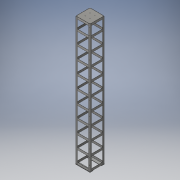
# Autodesk Inventor part: Celosia
Saved by Autodesk Inventor 2016 (Build 200138000, 138)
## iProperties
Created: 2017-01-18
Part Number: Celosia
Material: Generic
Document SubType Name: Modeling
Designer: admin
Density: 1 g/cm^3
Appearance: Default
Author: admin
Autodesk Inventor part; units mm, degrees
(part 1 of 3)
ref_plane "YZ Plane" through (0, 0, 0) normal (1, 0, 0) x (0, 1, 0)
ref_plane "XZ Plane" through (0, 0, 0) normal (0, 1, 0) x (-1, 0, 0)
ref_plane "XY Plane" through (0, 0, 0) normal (0, 0, 1) x (1, 0, 0)
sketch "Sketch1" plane through (0, 0, 0) normal (0, 1, 0) x (-1, 0, 0)
  line L0 (350, 345.4342) -> (345.4342, 350)
  line L1 (350, 320.2894) -> (342, 328.2894)
  line L2 (328.2894, 342) -> (320.2894, 350)
  line L3 (350, 295.1447) -> (342, 303.1447)
  line L4 (303.1447, 342) -> (295.1447, 350)
  line L5 (350, 270) -> (342, 278)
  line L6 (278, 342) -> (270, 350)
  line L7 (-270.2598, 345.6939) -> (-274.5658, 350)
  line L8 (-291.7106, 342) -> (-299.7106, 350)
  line L9 (-316.8553, 342) -> (-324.8553, 350)
  line L10 (-339.0697, 339.0697) -> (-350, 350)
  line L11 (-342, 316.8553) -> (-350, 324.8553)
  line L12 (-342, 291.7106) -> (-350, 299.7106)
  line L13 (-345.6939, 270.2598) -> (-350, 274.5658)
  line L14 (350, -273) -> (347, -270)
  line L15 (350, -298.1447) -> (342, -290.1447)
  line L16 (350, -323.2894) -> (342, -315.2894)
  line L17 (350, -348.4342) -> (339.6983, -338.1324)
  line L18 (326.4211, -350) -> (318.4211, -342)
  line L19 (301.2764, -350) -> (293.2764, -342)
  line L20 (276.1317, -350) -> (271.5658, -345.4342)
  line L21 (271.5658, -345.4342) -> (270.7161, -344.5844)
  line L22 (-270.3806, -345.0866) -> (-273.0153, -342.4519)
  line L23 (-342.4189, -273.0483) -> (-345.0146, -270.4526)
  line L24 (-290.6119, -350) -> (-298.6119, -342)
  line L25 (-342, -298.6119) -> (-350, -290.6119)
  line L26 (-315.7566, -350) -> (-323.7566, -342)
  line L27 (-342, -323.7566) -> (-350, -315.7566)
  line L28 (-340.9013, -350) -> (-350, -340.9013)
  line L29 (-310, 360) -> (-310, 342)
  line L30 (-319, 350) -> (-319, 342)
  line L31 (-301, 350) -> (-301, 342)
  line L32 (310, -360) -> (310, -342)
  line L33 (319, -350) -> (319, -342)
  line L34 (301, -350) -> (301, -342)
  line L35 (350, 270) -> (347, 270)
  line L36 (350, 350) -> (270, 350)
  line L37 (270, 350) -> (270, 347)
  line L38 (332, 342) -> (275, 342)
  line L39 (342, 332) -> (342, 275)
  line L40 (270, 347) -> (270.3806, 345.0866)
  line L41 (270.3806, 345.0866) -> (271.4645, 343.4645)
  line L42 (271.4645, 343.4645) -> (273.0866, 342.3806)
  line L43 (273.0866, 342.3806) -> (275, 342)
  line L44 (342, 275) -> (342.3806, 273.0866)
  line L45 (342.3806, 273.0866) -> (343.4645, 271.4645)
  line L46 (343.4645, 271.4645) -> (345.0866, 270.3806)
  line L47 (345.0866, 270.3806) -> (347, 270)
  line L48 (350, 350) -> (350, 270)
  line L49 (332, 342) -> (335.8268, 341.2388)
  arc A0 (341.2388, 335.8268) -> (335.8268, 341.2388) centre (332, 332) ccw
  line L50 (341.2388, 335.8268) -> (342, 332)
  line L51 (-347, 270) -> (-350, 270)
  line L52 (-270, 350) -> (-350, 350)
  line L53 (-350, 350) -> (-350, 270)
  line L54 (-347, 270) -> (-345.0866, 270.3806)
  line L55 (-345.0866, 270.3806) -> (-343.4645, 271.4645)
  line L56 (-343.4645, 271.4645) -> (-342.3806, 273.0866)
  line L57 (-342.3806, 273.0866) -> (-342, 275)
  line L58 (-275, 342) -> (-273.0866, 342.3806)
  line L59 (-273.0866, 342.3806) -> (-271.4645, 343.4645)
  line L60 (-271.4645, 343.4645) -> (-270.3806, 345.0866)
  line L61 (-270.3806, 345.0866) -> (-270, 347)
  line L62 (-270, 347) -> (-270, 350)
  line L63 (-275, 342) -> (-332, 342)
  line L64 (-342, 332) -> (-342, 275)
  line L65 (-342, 332) -> (-341.2388, 335.8268)
  arc A1 (-335.8268, 341.2388) -> (-341.2388, 335.8268) centre (-332, 332) ccw
  line L66 (-335.8268, 341.2388) -> (-332, 342)
  line L67 (270, 347) -> (270, 342)
  line L68 (-270, 347) -> (-270, 342)
  line L69 (-270, 342) -> (270, 342)
  line L70 (-270, 350) -> (270, 350)
  circle A2 centre (-330, -330) radius 7
  line L71 (-316, -330) -> (-344, -330)
  line L72 (-330, -316) -> (-330, -344)
  circle A3 centre (330, -330) radius 7
  line L73 (344, -330) -> (316, -330)
  line L74 (330, -316) -> (330, -344)
  circle A4 centre (-330, 330) radius 7
  line L75 (-316, 330) -> (-344, 330)
  line L76 (-330, 344) -> (-330, 316)
  circle A5 centre (330, 330) radius 7
  line L77 (344, 330) -> (316, 330)
  line L78 (330, 344) -> (330, 316)
  circle A6 centre (-270, 270) radius 13
  line L79 (-244, 270) -> (-296, 270)
  line L80 (-270, 296) -> (-270, 244)
  circle A7 centre (270, 270) radius 13
  line L81 (296, 270) -> (244, 270)
  line L82 (270, 296) -> (270, 244)
  circle A8 centre (-270, -270) radius 13
  line L83 (-244, -270) -> (-296, -270)
  line L84 (-270, -244) -> (-270, -296)
  circle A9 centre (270, -270) radius 13
  line L85 (296, -270) -> (244, -270)
  line L86 (270, -244) -> (270, -296)
  line L87 (360, 360) -> (360, 210)
  line L88 (360, 210) -> (350, 210)
  line L89 (342, 210) -> (-342, 210)
  line L90 (-360, 360) -> (-360, 210)
  line L91 (-360, 210) -> (-350, 210)
  line L92 (360, 360) -> (-360, 360)
  line L93 (360, -360) -> (-360, -360)
  line L94 (360, -210) -> (350, -210)
  line L95 (-360, -210) -> (-350, -210)
  line L96 (360, -210) -> (360, -360)
  line L97 (342, -210) -> (-342, -210)
  line L98 (-360, -210) -> (-360, -360)
  line L99 (350, -350) -> (270, -350)
  line L100 (350, -270) -> (347, -270)
  line L101 (342, -275) -> (342, -332)
  line L102 (332, -342) -> (275, -342)
  line L103 (270, -347) -> (270, -350)
  line L104 (347, -270) -> (345.0866, -270.3806)
  line L105 (345.0866, -270.3806) -> (343.4645, -271.4645)
  line L106 (343.4645, -271.4645) -> (342.3806, -273.0866)
  line L107 (342.3806, -273.0866) -> (342, -275)
  line L108 (275, -342) -> (273.0866, -342.3806)
  line L109 (273.0866, -342.3806) -> (271.4645, -343.4645)
  line L110 (271.4645, -343.4645) -> (270.3806, -345.0866)
  line L111 (270.3806, -345.0866) -> (270, -347)
  line L112 (350, -270) -> (350, -350)
  line L113 (342, -332) -> (341.2388, -335.8268)
  arc A10 (335.8268, -341.2388) -> (341.2388, -335.8268) centre (332, -332) ccw
  line L114 (335.8268, -341.2388) -> (332, -342)
  line L115 (-270, -350) -> (-350, -350)
  line L116 (-275, -342) -> (-332, -342)
  line L117 (-342, -275) -> (-342, -332)
  line L118 (-347, -270) -> (-350, -270)
  line L119 (-350, -270) -> (-350, -350)
  line L120 (-271.4645, -343.4645) -> (-273.0866, -342.3806)
  line L121 (-273.0866, -342.3806) -> (-275, -342)
  line L122 (-342, -275) -> (-342.3806, -273.0866)
  line L123 (-342.3806, -273.0866) -> (-343.4645, -271.4645)
  line L124 (-347, -270) -> (-345.0866, -270.3806)
  line L125 (-345.0866, -270.3806) -> (-343.4645, -271.4645)
  line L126 (-271.4645, -343.4645) -> (-270.3806, -345.0866)
  line L127 (-270.3806, -345.0866) -> (-270, -347)
  line L128 (-270, -347) -> (-270, -350)
  line L129 (-332, -342) -> (-335.8268, -341.2388)
  arc A11 (-341.2388, -335.8268) -> (-335.8268, -341.2388) centre (-332, -332) ccw
  line L130 (-341.2388, -335.8268) -> (-342, -332)
  line L131 (347, -270) -> (342, -270)
  line L132 (347, 270) -> (342, 270)
  line L133 (342, 270) -> (342, -270)
  line L134 (350, -270) -> (350, 270)
  line L135 (270, -350) -> (-270, -350)
  line L136 (-20, -350) -> (-20, -342)
  line L137 (20, -350) -> (20, -342)
  line L138 (270, -347) -> (270, -342)
  line L139 (270, -342) -> (-270, -342)
  line L140 (-270, -342) -> (-270, -347)
  line L141 (0, -350) -> (0, -342)
  line L142 (-342, 270) -> (-347, 270)
  line L143 (-342, -270) -> (-347, -270)
  line L144 (-342, 270) -> (-342, -270)
  line L145 (-350, 270) -> (-350, -270)
  line L146 (0, -360) -> (0, 360) construction
  line L147 (350, 0) -> (-350, 0) construction
  line L148 (360, -360) -> (-360, -360)
  line L149 (-360, -360) -> (-360, -210)
  line L150 (-360, -210) -> (360, -210)
  line L151 (360, -210) -> (360, -360)
  line L152 (360, 210) -> (-360, 210)
  line L153 (-360, 210) -> (-360, 360)
  line L154 (-360, 360) -> (360, 360)
  line L155 (360, 360) -> (360, 210)
  point P0 (0, 0)
  constraints: 312 end point, 70 point on line, 12 centre point, 8 point on circle, 6 midpoint, 4 parallel, 2 horizontal, 2 perpendicular
sketch "Sketch2" plane through (0, 0, 0) normal (0, 1, 0) x (-1, 0, 0)
  line L0 (-360, -360) -> (-360, -210) projected
  line L1 (-360, -210) -> (360, -210) projected
  line L2 (360, -360) -> (-360, -360) projected
  line L3 (360, -210) -> (360, -360) projected
  line L4 (360, 360) -> (360, 210) projected
  line L5 (360, 210) -> (-360, 210) projected
  line L6 (-360, 360) -> (360, 360) projected
  line L7 (-360, 210) -> (-360, 360) projected
  circle A0 centre (-330, 330) radius 7 projected
  circle A1 centre (-270, 270) radius 13 projected
  circle A2 centre (270, 270) radius 13 projected
  circle A3 centre (330, 330) radius 7 projected
  circle A4 centre (270, -270) radius 13 projected
  circle A5 centre (330, -330) radius 7 projected
  circle A6 centre (-270, -270) radius 13 projected
  point P0 (0, 0)
extrude "Extrusion1" add sketch "Sketch2" along normal blind 15
sketch "Sketch3" plane through (0, 15, 0) normal (0, 1, 0) x (1, 0, 0)
  line L0 (-350, -350) -> (-350, -270) projected
  line L1 (-350, -350) -> (-270, -350) projected
  line L2 (-270, -350) -> (-270, -347) projected
  line L3 (-270, -347) -> (-270.3806, -345.0866) projected
  line L4 (-332, -342) -> (-275, -342) projected
  arc A0 (-341.2388, -335.8268) -> (-335.8268, -341.2388) centre (-332, -332) ccw projected
  line L5 (-342, -332) -> (-342, -275) projected
  line L6 (-350, -270) -> (-347, -270) projected
  line L7 (-350, 270) -> (-347, 270) projected
  line L8 (-350, 270) -> (-350, 350) projected
  line L9 (-350, 350) -> (-270, 350) projected
  line L10 (-270, 347) -> (-270, 350) projected
  line L11 (-332, 342) -> (-275, 342) projected
  line L12 (-342, 275) -> (-342, 332) projected
  line L13 (350, 270) -> (350, 350) projected
  line L14 (270, 350) -> (350, 350) projected
  line L15 (275, 342) -> (332, 342) projected
  line L16 (342, 275) -> (342, 332) projected
  line L17 (347, 270) -> (350, 270) projected
  line L18 (270, 347) -> (270, 350) projected
  line L19 (350, -350) -> (350, -270) projected
  line L20 (342, -332) -> (342, -275) projected
  line L21 (275, -342) -> (332, -342) projected
  line L22 (270, -350) -> (350, -350) projected
  line L23 (270, -347) -> (270, -350) projected
  line L24 (347, -270) -> (350, -270) projected
  arc A1 (-270, -347) -> (-275, -342) centre (-275, -347) ccw
  arc A2 (-342, -332) -> (-332, -342) centre (-332, -332) ccw
  arc A3 (-342, -275) -> (-347, -270) centre (-347, -275) ccw
  arc A4 (-347, 270) -> (-342, 275) centre (-347, 275) ccw
  arc A5 (-332, 342) -> (-342, 332) centre (-331.75, 331.75) ccw
  arc A6 (-275, 342) -> (-270, 347) centre (-275, 347) ccw
  arc A7 (270, 347) -> (275, 342) centre (275, 347) ccw
  arc A8 (342, 332) -> (332, 342) centre (332, 332) ccw
  arc A9 (342, 275) -> (347, 270) centre (347, 275) ccw
  arc A10 (347, -270) -> (342, -275) centre (347, -275) ccw
  arc A11 (332, -342) -> (342, -332) centre (332, -332) ccw
  arc A12 (275, -342) -> (270, -347) centre (275, -347) ccw
  line L25 (-270, -347) -> (-270, -350)
  line L26 (-270, -350) -> (-350, -350)
  line L27 (-350, -270) -> (-350, -350)
  line L28 (-347, -270) -> (-350, -270)
  line L29 (-342, -275) -> (-342, -332)
  line L30 (-332, -342) -> (-275, -342)
  line L31 (-347, 270) -> (-350, 270)
  line L32 (-350, 270) -> (-350, 350)
  line L33 (-270, 350) -> (-350, 350)
  line L34 (-270, 350) -> (-270, 347)
  line L35 (-275, 342) -> (-332, 342)
  line L36 (-342, 332) -> (-342, 275)
  line L37 (270, 347) -> (270, 350)
  line L38 (270, 350) -> (350, 350)
  line L39 (350, 270) -> (350, 350)
  line L40 (350, 270) -> (347, 270)
  line L41 (342, 275) -> (342, 332)
  line L42 (332, 342) -> (275, 342)
  line L43 (347, -270) -> (350, -270)
  line L44 (350, -350) -> (350, -270)
  line L45 (350, -350) -> (270, -350)
  line L46 (270, -350) -> (270, -347)
  line L47 (275, -342) -> (332, -342)
  line L48 (342, -332) -> (342, -275)
  point P0 (0, 0)
  constraints: 48 end point, 25 point on circle, 12 centre point, 10 tangent, 9 perpendicular, 8 collinear, 2 parallel, 2 point on line, 1 concentric, 1 vertical
extrude "Extrusion2" add sketch "Sketch3" along normal blind 6390 separate body contours L0 L6 A3 L5 A2 A0 L4 A1 L3 L2 L1 | L3 A1
extrude "Extrusion3" add sketch "Sketch3" along normal blind 6390 separate body contours L22 L23 A12 L21 A11 L20 A10 L24 L19
extrude "Extrusion4" add sketch "Sketch3" along normal blind 6390 separate body contours L17 A9 L16 A8 L15 A7 L18 L14 L13
extrude "Extrusion5" add sketch "Sketch3" along normal blind 6390 separate body contours L8 L9 L10 A6 L11 A5 L12 A4 L7
sketch "Sketch4" plane through (-270, 15, 350) normal (0, 0, 1) x (1, 0, 0)
  arc A0 (-409.6145, 6425) -> (-409.6145, 6375) centre (-409.6145, 6400) ccw
  arc A1 (1027.0787, 6466.7022) -> (1027.0787, 6416.7022) centre (1027.0787, 6441.7022) ccw
  line L0 (-247.72, 0) -> (691.1461, 0)
  line L1 (726.1461, 0) -> (757.4906, 0)
  line L2 (-395.1565, -25) -> (-272.72, -25)
  line L3 (-395.1565, 25) -> (-272.72, 25)
  arc A2 (-272.72, -25) -> (-272.72, 25) centre (-272.72, 0) ccw
  arc A3 (-395.1565, 25) -> (-395.1565, -25) centre (-395.1565, 0) ccw
  line L4 (620, -156.6377) -> (620, -57.49)
  line L5 (620, -22.49) -> (620, 6494.5174)
  line L6 (605.0195, -206.6377) -> (634.9805, -206.6377)
  line L7 (605.0195, -156.6377) -> (634.9805, -156.6377)
  arc A4 (634.9805, -206.6377) -> (634.9805, -156.6377) centre (634.9805, -181.6377) ccw
  arc A5 (605.0195, -156.6377) -> (605.0195, -206.6377) centre (605.0195, -181.6377) ccw
  line L8 (270, -156.6377) -> (270, 6494.5174)
  line L9 (245.5273, -206.6377) -> (294.4727, -206.6377)
  line L10 (245.5273, -156.6377) -> (294.4727, -156.6377)
  arc A6 (294.4727, -206.6377) -> (294.4727, -156.6377) centre (294.4727, -181.6377) ccw
  arc A7 (245.5273, -156.6377) -> (245.5273, -206.6377) centre (245.5273, -181.6377) ccw
  line L11 (-80, -156.6377) -> (-80, 6494.5174)
  line L12 (-94.9805, -206.6377) -> (-65.0195, -206.6377)
  line L13 (-94.9805, -156.6377) -> (-65.0195, -156.6377)
  arc A8 (-65.0195, -206.6377) -> (-65.0195, -156.6377) centre (-65.0195, -181.6377) ccw
  arc A9 (-94.9805, -156.6377) -> (-94.9805, -206.6377) centre (-94.9805, -181.6377) ccw
  line L14 (-247.72, 6400) -> (741.1461, 6400)
  line L15 (-409.6145, 6375) -> (-272.72, 6375)
  line L16 (-409.6145, 6425) -> (-272.72, 6425)
  arc A10 (-272.72, 6375) -> (-272.72, 6425) centre (-272.72, 6400) ccw
  line L17 (738.6461, 75) -> (728.6461, 75)
  line L18 (733.6461, 100) -> (733.6461, 640)
  line L19 (550, 100) -> (753.6461, 100)
  line L20 (728.6461, 125) -> (733.6461, 100)
  line L21 (738.6461, 125) -> (733.6461, 100)
  line L22 (728.6461, 125) -> (738.6461, 125)
  line L23 (550, 640) -> (753.6461, 640)
  line L24 (738.6461, 615) -> (733.6461, 640)
  line L25 (728.6461, 615) -> (733.6461, 640)
  line L26 (738.6461, 615) -> (728.6461, 615)
  line L27 (733.6461, 640) -> (733.6461, 740)
  line L28 (550, 640) -> (753.6461, 640)
  line L29 (728.6461, 665) -> (733.6461, 640)
  line L30 (738.6461, 665) -> (733.6461, 640)
  line L31 (728.6461, 665) -> (738.6461, 665)
  line L32 (550, 740) -> (753.6461, 740)
  line L33 (738.6461, 715) -> (733.6461, 740)
  line L34 (728.6461, 715) -> (733.6461, 740)
  line L35 (738.6461, 715) -> (728.6461, 715)
  line L36 (733.6461, 740) -> (733.6461, 1280)
  line L37 (550, 740) -> (753.6461, 740)
  line L38 (728.6461, 765) -> (733.6461, 740)
  line L39 (738.6461, 765) -> (733.6461, 740)
  line L40 (728.6461, 765) -> (738.6461, 765)
  line L41 (550, 1280) -> (753.6461, 1280)
  line L42 (738.6461, 1255) -> (733.6461, 1280)
  line L43 (728.6461, 1255) -> (733.6461, 1280)
  line L44 (738.6461, 1255) -> (728.6461, 1255)
  line L45 (733.6461, 1280) -> (733.6461, 1380)
  line L46 (550, 1280) -> (753.6461, 1280)
  line L47 (728.6461, 1305) -> (733.6461, 1280)
  line L48 (738.6461, 1305) -> (733.6461, 1280)
  line L49 (728.6461, 1305) -> (738.6461, 1305)
  line L50 (550, 1380) -> (753.6461, 1380)
  line L51 (738.6461, 1355) -> (733.6461, 1380)
  line L52 (728.6461, 1355) -> (733.6461, 1380)
  line L53 (738.6461, 1355) -> (728.6461, 1355)
  line L54 (733.6461, 1380) -> (733.6461, 1920)
  line L55 (550, 1380) -> (753.6461, 1380)
  line L56 (728.6461, 1405) -> (733.6461, 1380)
  line L57 (738.6461, 1405) -> (733.6461, 1380)
  line L58 (728.6461, 1405) -> (738.6461, 1405)
  line L59 (550, 1920) -> (753.6461, 1920)
  line L60 (738.6461, 1895) -> (733.6461, 1920)
  line L61 (728.6461, 1895) -> (733.6461, 1920)
  line L62 (738.6461, 1895) -> (728.6461, 1895)
  line L63 (733.6461, 1920) -> (733.6461, 2020)
  line L64 (550, 1920) -> (753.6461, 1920)
  line L65 (728.6461, 1945) -> (733.6461, 1920)
  line L66 (738.6461, 1945) -> (733.6461, 1920)
  line L67 (728.6461, 1945) -> (738.6461, 1945)
  line L68 (550, 2020) -> (753.6461, 2020)
  line L69 (738.6461, 1995) -> (733.6461, 2020)
  line L70 (728.6461, 1995) -> (733.6461, 2020)
  line L71 (738.6461, 1995) -> (728.6461, 1995)
  line L72 (550, 2020) -> (753.6461, 2020)
  line L73 (728.6461, 2045) -> (733.6461, 2020)
  line L74 (738.6461, 2045) -> (733.6461, 2020)
  line L75 (728.6461, 2045) -> (738.6461, 2045)
  line L76 (550, 2560) -> (753.6461, 2560)
  line L77 (738.6461, 2535) -> (733.6461, 2560)
  line L78 (728.6461, 2535) -> (733.6461, 2560)
  line L79 (733.6461, 2020) -> (733.6461, 2560)
  line L80 (738.6461, 2535) -> (728.6461, 2535)
  line L81 (733.6461, 2560) -> (733.6461, 2660)
  line L82 (550, 2560) -> (753.6461, 2560)
  line L83 (728.6461, 2585) -> (733.6461, 2560)
  line L84 (738.6461, 2585) -> (733.6461, 2560)
  line L85 (728.6461, 2585) -> (738.6461, 2585)
  line L86 (550, 2660) -> (753.6461, 2660)
  line L87 (738.6461, 2635) -> (733.6461, 2660)
  line L88 (728.6461, 2635) -> (733.6461, 2660)
  line L89 (738.6461, 2635) -> (728.6461, 2635)
  line L90 (733.6461, 2660) -> (733.6461, 3200)
  line L91 (550, 2660) -> (753.6461, 2660)
  line L92 (728.6461, 2685) -> (733.6461, 2660)
  line L93 (738.6461, 2685) -> (733.6461, 2660)
  line L94 (728.6461, 2685) -> (738.6461, 2685)
  line L95 (550, 3200) -> (753.6461, 3200)
  line L96 (738.6461, 3175) -> (733.6461, 3200)
  line L97 (728.6461, 3175) -> (733.6461, 3200)
  line L98 (738.6461, 3175) -> (728.6461, 3175)
  line L99 (733.6461, 3200) -> (733.6461, 3300)
  line L100 (550, 3200) -> (753.6461, 3200)
  line L101 (728.6461, 3225) -> (733.6461, 3200)
  line L102 (738.6461, 3225) -> (733.6461, 3200)
  line L103 (728.6461, 3225) -> (738.6461, 3225)
  line L104 (550, 3300) -> (753.6461, 3300)
  line L105 (738.6461, 3275) -> (733.6461, 3300)
  line L106 (728.6461, 3275) -> (733.6461, 3300)
  line L107 (738.6461, 3275) -> (728.6461, 3275)
  line L108 (733.6461, 3300) -> (733.6461, 3840)
  line L109 (550, 3300) -> (753.6461, 3300)
  line L110 (728.6461, 3325) -> (733.6461, 3300)
  line L111 (738.6461, 3325) -> (733.6461, 3300)
  line L112 (728.6461, 3325) -> (738.6461, 3325)
  line L113 (550, 3840) -> (753.6461, 3840)
  line L114 (738.6461, 3815) -> (733.6461, 3840)
  line L115 (728.6461, 3815) -> (733.6461, 3840)
  line L116 (738.6461, 3815) -> (728.6461, 3815)
  line L117 (733.6461, 3840) -> (733.6461, 3940)
  line L118 (550, 3840) -> (753.6461, 3840)
  line L119 (728.6461, 3865) -> (733.6461, 3840)
  line L120 (738.6461, 3865) -> (733.6461, 3840)
  line L121 (728.6461, 3865) -> (738.6461, 3865)
  line L122 (550, 3940) -> (753.6461, 3940)
  line L123 (738.6461, 3915) -> (733.6461, 3940)
  line L124 (728.6461, 3915) -> (733.6461, 3940)
  line L125 (738.6461, 3915) -> (728.6461, 3915)
  line L126 (733.6461, 3940) -> (733.6461, 4480)
  line L127 (550, 3940) -> (753.6461, 3940)
  line L128 (728.6461, 3965) -> (733.6461, 3940)
  line L129 (738.6461, 3965) -> (733.6461, 3940)
  line L130 (728.6461, 3965) -> (738.6461, 3965)
  line L131 (550, 4480) -> (753.6461, 4480)
  line L132 (738.6461, 4455) -> (733.6461, 4480)
  line L133 (728.6461, 4455) -> (733.6461, 4480)
  line L134 (738.6461, 4455) -> (728.6461, 4455)
  line L135 (550, 4480) -> (753.6461, 4480)
  line L136 (728.6461, 4505) -> (733.6461, 4480)
  line L137 (738.6461, 4505) -> (733.6461, 4480)
  line L138 (728.6461, 4505) -> (738.6461, 4505)
  line L139 (550, 4580) -> (753.6461, 4580)
  line L140 (738.6461, 4555) -> (733.6461, 4580)
  line L141 (728.6461, 4555) -> (733.6461, 4580)
  line L142 (738.6461, 4555) -> (728.6461, 4555)
  line L143 (733.6461, 4580) -> (733.6461, 5120)
  line L144 (550, 4580) -> (753.6461, 4580)
  line L145 (728.6461, 4605) -> (733.6461, 4580)
  line L146 (738.6461, 4605) -> (733.6461, 4580)
  line L147 (728.6461, 4605) -> (738.6461, 4605)
  line L148 (550, 5120) -> (753.6461, 5120)
  line L149 (738.6461, 5095) -> (733.6461, 5120)
  line L150 (728.6461, 5095) -> (733.6461, 5120)
  line L151 (738.6461, 5095) -> (728.6461, 5095)
  line L152 (733.6461, 5120) -> (733.6461, 5220)
  line L153 (550, 5120) -> (753.6461, 5120)
  line L154 (728.6461, 5145) -> (733.6461, 5120)
  line L155 (738.6461, 5145) -> (733.6461, 5120)
  line L156 (728.6461, 5145) -> (738.6461, 5145)
  line L157 (550, 5220) -> (753.6461, 5220)
  line L158 (738.6461, 5195) -> (733.6461, 5220)
  line L159 (728.6461, 5195) -> (733.6461, 5220)
  line L160 (738.6461, 5195) -> (728.6461, 5195)
  line L161 (733.6461, 5220) -> (733.6461, 5760)
  line L162 (550, 5220) -> (753.6461, 5220)
  line L163 (728.6461, 5245) -> (733.6461, 5220)
  line L164 (738.6461, 5245) -> (733.6461, 5220)
  line L165 (728.6461, 5245) -> (738.6461, 5245)
  line L166 (550, 5760) -> (753.6461, 5760)
  line L167 (738.6461, 5735) -> (733.6461, 5760)
  line L168 (728.6461, 5735) -> (733.6461, 5760)
  line L169 (738.6461, 5735) -> (728.6461, 5735)
  line L170 (733.6461, 5760) -> (733.6461, 5860)
  line L171 (550, 5760) -> (753.6461, 5760)
  line L172 (728.6461, 5785) -> (733.6461, 5760)
  line L173 (738.6461, 5785) -> (733.6461, 5760)
  line L174 (728.6461, 5785) -> (738.6461, 5785)
  line L175 (550, 5860) -> (753.6461, 5860)
  line L176 (738.6461, 5835) -> (733.6461, 5860)
  line L177 (728.6461, 5835) -> (733.6461, 5860)
  line L178 (738.6461, 5835) -> (728.6461, 5835)
  line L179 (726.1461, 0) -> (753.6461, 0)
  line L180 (733.6461, 5860) -> (733.6461, 6290)
  line L181 (550, 5860) -> (753.6461, 5860)
  line L182 (728.6461, 5885) -> (733.6461, 5860)
  line L183 (738.6461, 5885) -> (733.6461, 5860)
  line L184 (728.6461, 5885) -> (738.6461, 5885)
  line L185 (550, 6290) -> (753.6461, 6290)
  line L186 (738.6461, 6265) -> (733.6461, 6290)
  line L187 (728.6461, 6265) -> (733.6461, 6290)
  line L188 (738.6461, 6265) -> (728.6461, 6265)
  line L189 (733.6461, 6290) -> (733.6461, 6390)
  line L190 (550, 6290) -> (753.6461, 6290)
  line L191 (728.6461, 6315) -> (733.6461, 6290)
  line L192 (738.6461, 6315) -> (733.6461, 6290)
  line L193 (728.6461, 6315) -> (738.6461, 6315)
  line L194 (630, 6390) -> (741.1461, 6390)
  line L195 (738.6461, 6365) -> (733.6461, 6390)
  line L196 (728.6461, 6365) -> (733.6461, 6390)
  line L197 (738.6461, 6365) -> (728.6461, 6365)
  line L198 (733.6461, -15) -> (733.6461, 0)
  line L199 (-5, -15) -> (753.6461, -15)
  line L200 (738.6461, -40) -> (733.6461, -15)
  line L201 (728.6461, -40) -> (733.6461, -15)
  line L202 (738.6461, -40) -> (728.6461, -40)
  line L203 (630, 0) -> (753.6461, 0)
  line L204 (728.6461, 25) -> (733.6461, 0)
  line L205 (738.6461, 25) -> (733.6461, 0)
  line L206 (728.6461, 25) -> (738.6461, 25)
  line L207 (733.6461, -15) -> (733.6461, -40)
  line L208 (733.6461, 0) -> (733.6461, 25)
  line L209 (733.6461, 6390) -> (733.6461, 6400)
  line L210 (630, 6390) -> (758.6461, 6390)
  line L211 (738.6461, 6365) -> (733.6461, 6390)
  line L212 (728.6461, 6365) -> (733.6461, 6390)
  line L213 (738.6461, 6365) -> (728.6461, 6365)
  line L214 (630, 6400) -> (758.6461, 6400)
  line L215 (728.6461, 6425) -> (733.6461, 6400)
  line L216 (738.6461, 6425) -> (733.6461, 6400)
  line L217 (728.6461, 6425) -> (738.6461, 6425)
  line L218 (733.6461, 6390) -> (733.6461, 6365)
  line L219 (733.6461, 6400) -> (733.6461, 6425)
  line L220 (831.2118, 0) -> (831.2118, 6400)
  line L221 (630, 0) -> (691.1461, 0)
  line L222 (726.1461, 0) -> (851.2118, 0)
  line L223 (826.2118, 25) -> (831.2118, 0)
  line L224 (836.2118, 25) -> (831.2118, 0)
  line L225 (826.2118, 25) -> (836.2118, 25)
  line L226 (630, 6400) -> (741.1461, 6400)
  line L227 (776.1461, 6400) -> (851.2118, 6400)
  line L228 (836.2118, 6375) -> (831.2118, 6400)
  line L229 (826.2118, 6375) -> (831.2118, 6400)
  line L230 (836.2118, 6375) -> (826.2118, 6375)
  line L231 (-80, 6491.9106) -> (620, 6491.9106)
  line L232 (-80, 6410) -> (-80, 6516.9106)
  line L233 (-55, 6496.9106) -> (-80, 6491.9106)
  line L234 (-55, 6486.9106) -> (-80, 6491.9106)
  line L235 (-55, 6496.9106) -> (-55, 6486.9106)
  line L236 (620, 6410) -> (620, 6516.9106)
  line L237 (595, 6486.9106) -> (620, 6491.9106)
  line L238 (595, 6496.9106) -> (620, 6491.9106)
  line L239 (595, 6486.9106) -> (595, 6496.9106)
  line L240 (733.6461, 0) -> (733.6461, 100)
  line L241 (630, 0) -> (691.1461, 0)
  line L242 (733.6461, 4480) -> (733.6461, 4580)
  line L243 (728.6461, 25) -> (733.6461, 0)
  line L244 (738.6461, 25) -> (733.6461, 0)
  line L245 (728.6461, 25) -> (738.6461, 25)
  line L246 (550, 100) -> (753.6461, 100)
  line L247 (738.6461, 75) -> (733.6461, 100)
  line L248 (728.6461, 75) -> (733.6461, 100)
  line L249 (-80, 5166) -> (-72, 5166)
  line L250 (480, 0) -> (60, 0)
  line L251 (540, 6390) -> (620, 6390)
  line L252 (620, 6390) -> (620, 0)
  line L253 (540, 0) -> (540, 6390)
  line L254 (-90, 270) -> (-72, 270)
  line L255 (-80, 279) -> (-72, 279)
  line L256 (-80, 261) -> (-72, 261)
  line L257 (0, 5120) -> (0, 5220)
  line L258 (0, 5220) -> (540, 5220)
  line L259 (540, 5220) -> (540, 5120)
  line L260 (540, 5120) -> (0, 5120)
  line L261 (0, 3840) -> (0, 3940)
  line L262 (540, 3200) -> (0, 3200)
  line L263 (540, 3300) -> (540, 3200)
  line L264 (0, 3300) -> (540, 3300)
  line L265 (0, 100) -> (540, 100)
  line L266 (0, 3200) -> (0, 3300)
  line L267 (540, 2560) -> (0, 2560)
  line L268 (540, 2660) -> (540, 2560)
  line L269 (0, 5760) -> (0, 5860)
  line L270 (0, 5860) -> (540, 5860)
  line L271 (540, 5860) -> (540, 5760)
  line L272 (540, 5760) -> (0, 5760)
  line L273 (0, 2660) -> (540, 2660)
  line L274 (0, 2560) -> (0, 2660)
  line L275 (540, 640) -> (0, 640)
  line L276 (540, 740) -> (540, 640)
  line L277 (0, 740) -> (540, 740)
  line L278 (0, 640) -> (0, 740)
  line L279 (0, 15) -> (0, -15)
  line L280 (-13, 0) -> (-13, -15)
  line L281 (600, 8) -> (600, -15)
  line L282 (593, 0) -> (593, -15)
  line L283 (607, 0) -> (607, -15)
  line L284 (540, 15) -> (540, -15)
  line L285 (527, 0) -> (527, -15)
  line L286 (553, 0) -> (553, -15)
  line L287 (630, -15) -> (630, 0)
  line L288 (630, 0) -> (480, 0)
  line L289 (480, 0) -> (480, -15)
  line L290 (480, -15) -> (630, -15)
  line L291 (-84, 620) -> (-72, 620)
  line L292 (-80, 624) -> (-72, 624)
  line L293 (-80, 616) -> (-72, 616)
  line L294 (-84, 970) -> (-72, 970)
  line L295 (-80, 974) -> (-72, 974)
  line L296 (-80, 966) -> (-72, 966)
  line L297 (-84, 1320) -> (-72, 1320)
  line L298 (-80, 1324) -> (-72, 1324)
  line L299 (-80, 1316) -> (-72, 1316)
  line L300 (-84, 1670) -> (-72, 1670)
  line L301 (-80, 1674) -> (-72, 1674)
  line L302 (-80, 1666) -> (-72, 1666)
  line L303 (-84, 2020) -> (-72, 2020)
  line L304 (-80, 2024) -> (-72, 2024)
  line L305 (-80, 2016) -> (-72, 2016)
  line L306 (-84, 2370) -> (-72, 2370)
  line L307 (-80, 2374) -> (-72, 2374)
  line L308 (-80, 2366) -> (-72, 2366)
  line L309 (-84, 2720) -> (-72, 2720)
  line L310 (-80, 2724) -> (-72, 2724)
  line L311 (-80, 2716) -> (-72, 2716)
  line L312 (-84, 3070) -> (-72, 3070)
  line L313 (-80, 3074) -> (-72, 3074)
  line L314 (-80, 3066) -> (-72, 3066)
  line L315 (-84, 3420) -> (-72, 3420)
  line L316 (-80, 3424) -> (-72, 3424)
  line L317 (-80, 3416) -> (-72, 3416)
  line L318 (-84, 3770) -> (-72, 3770)
  line L319 (-80, 3774) -> (-72, 3774)
  line L320 (-80, 3766) -> (-72, 3766)
  line L321 (-84, 4120) -> (-72, 4120)
  line L322 (-80, 4124) -> (-72, 4124)
  line L323 (-80, 4116) -> (-72, 4116)
  line L324 (-84, 4470) -> (-72, 4470)
  line L325 (-80, 4474) -> (-72, 4474)
  line L326 (-80, 4466) -> (-72, 4466)
  line L327 (-84, 4820) -> (-72, 4820)
  line L328 (-80, 4824) -> (-72, 4824)
  line L329 (-80, 4816) -> (-72, 4816)
  line L330 (-84, 5170) -> (-72, 5170)
  line L331 (-80, 5174) -> (-72, 5174)
  line L332 (-84, 5520) -> (-72, 5520)
  line L333 (-80, 5524) -> (-72, 5524)
  line L334 (-80, 5516) -> (-72, 5516)
  line L335 (-84, 5870) -> (-72, 5870)
  line L336 (-80, 5874) -> (-72, 5874)
  line L337 (-80, 5866) -> (-72, 5866)
  line L338 (-84, 6220) -> (-72, 6220)
  line L339 (-80, 6224) -> (-72, 6224)
  line L340 (-80, 6216) -> (-72, 6216)
  line L341 (0, 1280) -> (0, 1380)
  line L342 (0, 1380) -> (540, 1380)
  line L343 (540, 1380) -> (540, 1280)
  line L344 (540, 1280) -> (0, 1280)
  line L345 (13, 0) -> (13, -15)
  line L346 (-60, 8) -> (-60, -15)
  line L347 (-67, 0) -> (-67, -15)
  line L348 (-53, 0) -> (-53, -15)
  line L349 (540, 100) -> (540, 0)
  line L350 (-90, -15) -> (60, -15)
  line L351 (60, -15) -> (60, 0)
  line L352 (60, 0) -> (-90, 0)
  line L353 (0, 1920) -> (0, 2020)
  line L354 (0, 2020) -> (540, 2020)
  line L355 (540, 2020) -> (540, 1920)
  line L356 (540, 1920) -> (0, 1920)
  line L357 (-80, 0) -> (-80, 6390)
  line L358 (-80, 6390) -> (0, 6390)
  line L359 (0, 6390) -> (0, 0)
  line L360 (0, 100) -> (0, 0)
  line L361 (0, 3940) -> (540, 3940)
  line L362 (540, 3940) -> (540, 3840)
  line L363 (540, 3840) -> (0, 3840)
  line L364 (0, 6290) -> (0, 6390)
  line L365 (0, 6390) -> (540, 6390)
  line L366 (540, 6390) -> (540, 6290)
  line L367 (540, 6290) -> (0, 6290)
  line L368 (580, 6390) -> (580, 6400)
  line L369 (620, 6400) -> (-80, 6400)
  line L370 (-40, 6390) -> (-40, 6400)
  line L371 (620, 6400) -> (620, 6390)
  line L372 (580, 6390) -> (-40, 6390)
  line L373 (-80, 6390) -> (-80, 6400)
  line L374 (0, 4480) -> (0, 4580)
  line L375 (0, 4580) -> (540, 4580)
  line L376 (540, 4580) -> (540, 4480)
  line L377 (540, 4480) -> (0, 4480)
  line L378 (-90, 0) -> (-90, -15)
  line L379 (-72, 5760) -> (-72, 5860)
  line L380 (612, 5760) -> (620, 5760)
  line L381 (620, 5760) -> (620, 5860)
  line L382 (620, 5860) -> (612, 5860)
  line L383 (612, 5860) -> (612, 5760)
  line L384 (-72, 1380) -> (-80, 1380)
  line L385 (-80, 1380) -> (-80, 1280)
  line L386 (-80, 1280) -> (-72, 1280)
  line L387 (-72, 1280) -> (-72, 1380)
  line L388 (612, 1280) -> (620, 1280)
  line L389 (620, 1280) -> (620, 1380)
  line L390 (620, 1380) -> (612, 1380)
  line L391 (612, 1380) -> (612, 1280)
  line L392 (-72, 2020) -> (-80, 2020)
  line L393 (-80, 2020) -> (-80, 1920)
  line L394 (-80, 1920) -> (-72, 1920)
  line L395 (-72, 1920) -> (-72, 2020)
  line L396 (612, 1920) -> (620, 1920)
  line L397 (620, 1920) -> (620, 2020)
  line L398 (620, 2020) -> (612, 2020)
  line L399 (612, 2020) -> (612, 1920)
  line L400 (612, 0) -> (620, 0)
  line L401 (-72, 4580) -> (-80, 4580)
  line L402 (0, 0) -> (-80, 0)
  line L403 (-72, 6390) -> (-72, 0)
  line L404 (612, 6390) -> (612, 0)
  line L405 (620, 0) -> (540, 0)
  line L406 (540, 0) -> (480, 0)
  line L407 (60, 0) -> (0, 0)
  line L408 (-72, 100) -> (-80, 100)
  line L409 (-80, 100) -> (-80, 0)
  line L410 (-80, 0) -> (-72, 0)
  line L411 (-72, 0) -> (-72, 100)
  line L412 (620, 3200) -> (620, 3300)
  line L413 (620, 0) -> (620, 100)
  line L414 (620, 100) -> (612, 100)
  line L415 (612, 100) -> (612, 0)
  line L416 (-72, 740) -> (-80, 740)
  line L417 (-80, 740) -> (-80, 640)
  line L418 (-80, 640) -> (-72, 640)
  line L419 (-72, 640) -> (-72, 740)
  line L420 (612, 640) -> (620, 640)
  line L421 (620, 640) -> (620, 740)
  line L422 (620, 740) -> (612, 740)
  line L423 (612, 740) -> (612, 640)
  line L424 (-72, 2660) -> (-80, 2660)
  line L425 (-80, 2660) -> (-80, 2560)
  line L426 (-80, 2560) -> (-72, 2560)
  line L427 (-72, 2560) -> (-72, 2660)
  line L428 (612, 2560) -> (620, 2560)
  line L429 (620, 2560) -> (620, 2660)
  line L430 (620, 2660) -> (612, 2660)
  line L431 (612, 2660) -> (612, 2560)
  line L432 (-72, 3300) -> (-80, 3300)
  line L433 (-80, 3300) -> (-80, 3200)
  line L434 (-80, 3200) -> (-72, 3200)
  line L435 (-72, 3200) -> (-72, 3300)
  line L436 (612, 3200) -> (620, 3200)
  line L437 (620, 3300) -> (612, 3300)
  line L438 (612, 3300) -> (612, 3200)
  line L439 (-80, 4580) -> (-80, 4480)
  line L440 (-80, 4480) -> (-72, 4480)
  line L441 (-72, 4480) -> (-72, 4580)
  line L442 (-72, 3940) -> (-80, 3940)
  line L443 (-80, 3940) -> (-80, 3840)
  line L444 (-80, 3840) -> (-72, 3840)
  line L445 (-72, 3840) -> (-72, 3940)
  line L446 (612, 3840) -> (620, 3840)
  line L447 (620, 3840) -> (620, 3940)
  line L448 (620, 3940) -> (612, 3940)
  line L449 (612, 4480) -> (620, 4480)
  line L450 (620, 4480) -> (620, 4580)
  line L451 (620, 4580) -> (612, 4580)
  line L452 (612, 4580) -> (612, 4480)
  line L453 (-72, 6390) -> (-80, 6390)
  line L454 (-80, 6390) -> (-80, 6290)
  line L455 (-80, 6290) -> (-72, 6290)
  line L456 (-72, 6290) -> (-72, 6390)
  line L457 (612, 6290) -> (620, 6290)
  line L458 (620, 6290) -> (620, 6390)
  line L459 (620, 6390) -> (612, 6390)
  line L460 (612, 6390) -> (612, 6290)
  line L461 (-72, 5220) -> (-80, 5220)
  line L462 (-80, 5220) -> (-80, 5120)
  line L463 (-80, 5120) -> (-72, 5120)
  line L464 (-72, 5120) -> (-72, 5220)
  line L465 (612, 5120) -> (620, 5120)
  line L466 (620, 5120) -> (620, 5220)
  line L467 (620, 6390) -> (580, 6390)
  line L468 (-40, 6390) -> (-80, 6390)
  line L469 (620, 5220) -> (612, 5220)
  line L470 (612, 5220) -> (612, 5120)
  line L471 (-72, 5860) -> (-80, 5860)
  line L472 (-80, 5860) -> (-80, 5760)
  line L473 (-80, 5760) -> (-72, 5760)
  line L474 (612, 3940) -> (612, 3840)
  line L475 (-170.2013, 6435) -> (-191.2013, 6435)
  line L476 (-180.7014, 6400) -> (-191.2013, 6435)
  line L477 (947.1369, 6399.9999) -> (889.3869, 6400.0001)
  line L478 (924.3869, 6400) -> (913.887, 6435)
  line L479 (924.3869, 6400) -> (934.887, 6435)
  line L480 (-180.7014, 6400) -> (-170.2013, 6435)
  line L481 (924.3869, 6500) -> (924.3869, 6400)
  line L482 (-180.7014, 6500) -> (-180.7014, 6400)
  line L483 (934.887, 6435) -> (913.887, 6435)
  line L484 (-145.7014, 6399.9999) -> (-203.4514, 6400.0001)
  line L485 (97.1439, 6601.0745) -> (441.7924, 6601.0745)
  line L486 (62.5, 2058) -> (165.2959, 2058)
  arc A11 (165.2959, 2021) -> (165.2959, 2058) centre (165.2959, 2039.5) ccw
  arc A12 (62.5, 2058) -> (62.5, 2021) centre (62.5, 2039.5) ccw
  line L487 (52.5, 1381) -> (155.2959, 1381)
  line L488 (52.5, 1418) -> (155.2959, 1418)
  arc A13 (155.2959, 1381) -> (155.2959, 1418) centre (155.2959, 1399.5) ccw
  arc A14 (52.5, 1418) -> (52.5, 1381) centre (52.5, 1399.5) ccw
  line L489 (538.578, -58.49) -> (641.3739, -58.49)
  line L490 (538.578, -21.49) -> (641.3739, -21.49)
  arc A15 (641.3739, -58.49) -> (641.3739, -21.49) centre (641.3739, -39.99) ccw
  arc A16 (538.578, -21.49) -> (538.578, -58.49) centre (538.578, -39.99) ccw
  line L491 (510.294, -11.706) -> (538.578, -21.49)
  line L492 (38, 5433.9579) -> (38, 5527.5253)
  line L493 (1, 5433.9579) -> (1, 5527.5253)
  arc A17 (38, 5527.5253) -> (1, 5527.5253) centre (19.5, 5527.5253) ccw
  arc A18 (1, 5433.9579) -> (38, 5433.9579) centre (19.5, 5433.9579) ccw
  line L494 (82.578, -58.49) -> (185.3739, -58.49)
  line L495 (82.578, -21.49) -> (185.3739, -21.49)
  arc A19 (185.3739, -58.49) -> (185.3739, -21.49) centre (185.3739, -39.99) ccw
  arc A20 (82.578, -21.49) -> (82.578, -58.49) centre (82.578, -39.99) ccw
  line L496 (54.294, -11.706) -> (82.578, -21.49)
  line L497 (539, 5429.668) -> (539, 5523.2354)
  line L498 (502, 5429.668) -> (502, 5523.2354)
  arc A21 (539, 5523.2354) -> (502, 5523.2354) centre (520.5, 5523.2354) ccw
  arc A22 (502, 5429.668) -> (539, 5429.668) centre (520.5, 5429.668) ccw
  line L499 (43.2288, 101) -> (146.0247, 101)
  line L500 (43.2288, 138) -> (146.0247, 138)
  arc A23 (146.0247, 101) -> (146.0247, 138) centre (146.0247, 119.5) ccw
  arc A24 (43.2288, 138) -> (43.2288, 101) centre (43.2288, 119.5) ccw
  line L501 (43.2288, 741) -> (146.0247, 741)
  line L502 (43.2288, 778) -> (146.0247, 778)
  arc A25 (146.0247, 741) -> (146.0247, 778) centre (146.0247, 759.5) ccw
  line L503 (62.5, 2021) -> (165.2959, 2021)
  line L504 (52.5, 5861) -> (155.2959, 5861)
  line L505 (52.5, 5898) -> (155.2959, 5898)
  arc A26 (155.2959, 5861) -> (155.2959, 5898) centre (155.2959, 5879.5) ccw
  arc A27 (52.5, 5898) -> (52.5, 5861) centre (52.5, 5879.5) ccw
  line L506 (52.5, 5221) -> (155.2959, 5221)
  line L507 (52.5, 5258) -> (155.2959, 5258)
  arc A28 (155.2959, 5221) -> (155.2959, 5258) centre (155.2959, 5239.5) ccw
  arc A29 (52.5, 5258) -> (52.5, 5221) centre (52.5, 5239.5) ccw
  line L508 (52.5, 4581) -> (155.2959, 4581)
  line L509 (52.5, 4618) -> (155.2959, 4618)
  arc A30 (155.2959, 4581) -> (155.2959, 4618) centre (155.2959, 4599.5) ccw
  arc A31 (52.5, 4618) -> (52.5, 4581) centre (52.5, 4599.5) ccw
  line L510 (88.578, 6407.49) -> (191.3739, 6407.49)
  line L511 (88.578, 6444.49) -> (191.3739, 6444.49)
  arc A32 (191.3739, 6407.49) -> (191.3739, 6444.49) centre (191.3739, 6425.99) ccw
  arc A33 (88.578, 6444.49) -> (88.578, 6407.49) centre (88.578, 6425.99) ccw
  line L512 (60.294, 6397.706) -> (88.578, 6407.49)
  line L513 (133.294, 6248.494) -> (236.0899, 6248.494)
  line L514 (133.294, 6285.494) -> (236.0899, 6285.494)
  arc A34 (236.0899, 6248.494) -> (236.0899, 6285.494) centre (236.0899, 6266.994) ccw
  arc A35 (133.294, 6285.494) -> (133.294, 6248.494) centre (133.294, 6266.994) ccw
  line L515 (108.294, 6310.294) -> (133.294, 6285.494)
  line L516 (52.5, 3941) -> (155.2959, 3941)
  line L517 (52.5, 3978) -> (155.2959, 3978)
  arc A36 (155.2959, 3941) -> (155.2959, 3978) centre (155.2959, 3959.5) ccw
  arc A37 (52.5, 3978) -> (52.5, 3941) centre (52.5, 3959.5) ccw
  line L518 (52.5, 3301) -> (155.2959, 3301)
  line L519 (52.5, 3338) -> (155.2959, 3338)
  arc A38 (155.2959, 3301) -> (155.2959, 3338) centre (155.2959, 3319.5) ccw
  arc A39 (52.5, 3338) -> (52.5, 3301) centre (52.5, 3319.5) ccw
  line L520 (52.5, 2661) -> (155.2959, 2661)
  line L521 (52.5, 2698) -> (155.2959, 2698)
  arc A40 (155.2959, 2661) -> (155.2959, 2698) centre (155.2959, 2679.5) ccw
  arc A41 (52.5, 2698) -> (52.5, 2661) centre (52.5, 2679.5) ccw
  arc A42 (43.2288, 778) -> (43.2288, 741) centre (43.2288, 759.5) ccw
  line L522 (-90, 0) -> (630, 0) projected
  line L523 (-80, 0) -> (-80, 6390) projected
  point P0 (270, -15)
  point P1 (-385.1565, -15)
  point P2 (615.0195, -196.6377)
  point P3 (255.5273, -196.6377)
  point P4 (-84.9805, -196.6377)
  point P5 (-399.6145, 6385)
  point P6 (721.1461, 22.1863)
  point P7 (721.1461, 342.1863)
  point P8 (721.1461, 662.1863)
  point P9 (721.1461, 982.1863)
  point P10 (721.1461, 1302.1863)
  point P11 (721.1461, 1622.1863)
  point P12 (721.1461, 1942.1863)
  point P13 (721.1461, 2262.1863)
  point P14 (721.1461, 2582.1863)
  point P15 (721.1461, 2902.1863)
  point P16 (721.1461, 3222.1863)
  point P17 (721.1461, 3542.1863)
  point P18 (721.1461, 3862.1863)
  point P19 (721.1461, 4182.1863)
  point P20 (721.1461, 4502.1863)
  point P21 (721.1461, 4822.1863)
  point P22 (721.1461, 5142.1863)
  point P23 (721.1461, 5462.1863)
  point P24 (721.1461, 5782.1863)
  point P25 (721.1461, 6047.1863)
  point P26 (721.1461, 6312.1863)
  point P27 (721.1461, -26.0425)
  point P28 (771.1461, 6376.4575)
  point P29 (818.7118, 3144.3848)
  point P30 (242.1863, 6504.4106)
  point P31 (-160.7014, 6450)
  point P32 (870.7541, 6450)
  point P33 (239.3107, 6568.5745)
  point P34 (97.1439, 6608.5745)
  point P35 (58.5, 1387)
  point P36 (544.578, -52.49)
  point P37 (32, 5439.9579)
  point P38 (88.578, -52.49)
  point P39 (533, 5435.668)
  point P40 (49.2288, 107)
  point P41 (49.2288, 747)
  point P42 (68.5, 2027)
  point P43 (58.5, 5867)
  point P44 (58.5, 5227)
  point P45 (58.5, 4587)
  point P46 (94.578, 6413.49)
  point P47 (139.294, 6254.494)
  point P48 (58.5, 3947)
  point P49 (58.5, 3307)
  point P50 (58.5, 2667)
  constraints: 1016 end point, 183 point on line, 88 point on circle, 43 centre point, 14 midpoint, 447 other
sketch "Sketch5" plane through (-270, 15, 350) normal (0, 0, 1) x (1, 0, 0)
  line L0 (0, 100) -> (540, 100) projected
  line L1 (-90, 0) -> (630, 0) projected
  line L2 (540, 0) -> (540, 6390) projected
  line L3 (0, 0) -> (0, 6390) projected
  line L4 (540, 640) -> (0, 640) projected
  line L5 (0, 740) -> (540, 740) projected
  line L6 (540, 1280) -> (0, 1280) projected
  line L7 (0, 1380) -> (540, 1380) projected
  line L8 (540, 1920) -> (0, 1920) projected
  line L9 (0, 2020) -> (540, 2020) projected
  line L10 (540, 2560) -> (0, 2560) projected
  line L11 (0, 2660) -> (540, 2660) projected
  line L12 (540, 3200) -> (0, 3200) projected
  line L13 (0, 3300) -> (540, 3300) projected
  line L14 (540, 3840) -> (0, 3840) projected
  line L15 (0, 3940) -> (540, 3940) projected
  line L16 (540, 4480) -> (0, 4480) projected
  line L17 (0, 4580) -> (540, 4580) projected
  line L18 (540, 5120) -> (0, 5120) projected
  line L19 (0, 5220) -> (540, 5220) projected
  line L20 (540, 5760) -> (0, 5760) projected
  line L21 (0, 5860) -> (540, 5860) projected
  line L22 (540, 6290) -> (0, 6290) projected
  line L23 (0, 6390) -> (540, 6390) projected
  line L24 (540, 100) -> (0, 100)
  line L25 (0, 100) -> (0, 0)
  line L26 (0, 0) -> (540, 0)
  line L27 (540, 0) -> (540, 100)
  line L28 (0, 740) -> (540, 740)
  line L29 (540, 740) -> (540, 640)
  line L30 (540, 640) -> (0, 640)
  line L31 (0, 640) -> (0, 740)
  line L32 (540, 1280) -> (0, 1280)
  line L33 (0, 1280) -> (0, 1380)
  line L34 (0, 1380) -> (540, 1380)
  line L35 (540, 1380) -> (540, 1280)
  line L36 (540, 1920) -> (0, 1920)
  line L37 (0, 1920) -> (0, 2020)
  line L38 (0, 2020) -> (540, 2020)
  line L39 (540, 2020) -> (540, 1920)
  line L40 (540, 2560) -> (0, 2560)
  line L41 (0, 2560) -> (0, 2660)
  line L42 (0, 2660) -> (540, 2660)
  line L43 (540, 2660) -> (540, 2560)
  line L44 (540, 3200) -> (0, 3200)
  line L45 (0, 3200) -> (0, 3300)
  line L46 (0, 3300) -> (540, 3300)
  line L47 (540, 3300) -> (540, 3200)
  line L48 (540, 3840) -> (0, 3840)
  line L49 (0, 3840) -> (0, 3940)
  line L50 (0, 3940) -> (540, 3940)
  line L51 (540, 3940) -> (540, 3840)
  line L52 (540, 4480) -> (0, 4480)
  line L53 (0, 4480) -> (0, 4580)
  line L54 (0, 4580) -> (540, 4580)
  line L55 (540, 4580) -> (540, 4480)
  line L56 (540, 5120) -> (0, 5120)
  line L57 (0, 5120) -> (0, 5220)
  line L58 (0, 5220) -> (540, 5220)
  line L59 (540, 5220) -> (540, 5120)
  line L60 (540, 5760) -> (0, 5760)
  line L61 (0, 5760) -> (0, 5860)
  line L62 (0, 5860) -> (540, 5860)
  line L63 (540, 5860) -> (540, 5760)
  line L64 (0, 6290) -> (540, 6290)
  line L65 (540, 6290) -> (540, 6390)
  line L66 (540, 6390) -> (0, 6390)
  line L67 (0, 6390) -> (0, 6290)
  point P0 (270, -15)
  constraints: 88 end point, 22 parallel, 11 horizontal, 11 perpendicular, 2 other
extrude "Extrusion6" add sketch "Sketch5" against normal blind 8 separate body contours L0 L2 L1 L3
extrude "Extrusion7" add sketch "Sketch5" against normal blind 8 separate body contours L3 L5 L2 L4
extrude "Extrusion8" add sketch "Sketch5" against normal blind 8 separate body contours L3 L7 L2 L6
extrude "Extrusion9" add sketch "Sketch5" against normal blind 8 separate body contours L3 L9 L2 L8
extrude "Extrusion10" add sketch "Sketch5" against normal blind 8 separate body contours L3 L11 L2 L10
extrude "Extrusion11" add sketch "Sketch5" against normal blind 8 separate body contours L3 L13 L2 L12
extrude "Extrusion12" add sketch "Sketch5" against normal blind 8 separate body contours L3 L15 L2 L14
extrude "Extrusion13" add sketch "Sketch5" against normal blind 8 separate body contours L3 L17 L2 L16
extrude "Extrusion14" add sketch "Sketch5" against normal blind 8 separate body contours L3 L19 L2 L18
extrude "Extrusion15" add sketch "Sketch5" against normal blind 8 separate body contours L3 L21 L2 L20
extrude "Extrusion16" add sketch "Sketch5" against normal blind 8 separate body contours L3 L23 L2 L22
pattern_circular "Circular Pattern1" count 4 over 360 about axis through (0, -10, 0) along (0, 1, 0) of "Extrusion16", "Extrusion15", "Extrusion14", "Extrusion13", "Extrusion12", "Extrusion11", "Extrusion10", "Extrusion9", "Extrusion8", "Extrusion7", "Extrusion6" bodies 16